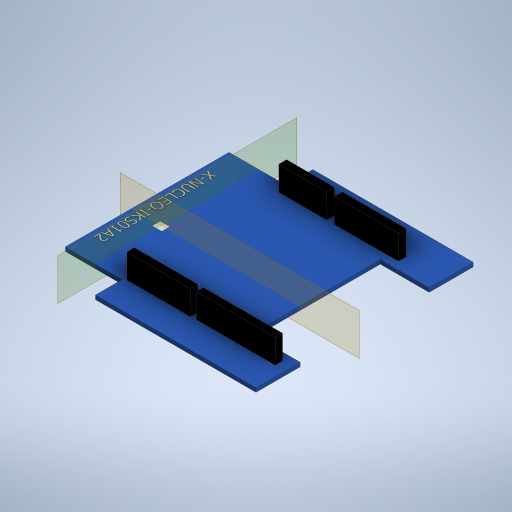
# Autodesk Inventor part: iks01A2base
Saved by Autodesk Inventor 2023 (Build 270158000, 158)
## iProperties
Created: 2023-11-05
Part Number: iks01A2base
Material: Générique
Document SubType Name: Modeling
Designer: eleves
Density: 1 g/cm^3
Appearance: Par défaut
Author: eleves
Autodesk Inventor part; units mm, degrees
ref_plane "YZ Plane" through (0, 0, 0) normal (1, 0, 0) x (0, 1, 0)
ref_plane "XZ Plane" through (0, 0, 0) normal (0, 1, 0) x (-1, 0, 0)
ref_plane "XY Plane" through (0, 0, 0) normal (0, 0, 1) x (1, 0, 0)
sketch "Esquisse1" plane through (0, 0, 0) normal (0, 1, 0) x (-1, 0, 0)
  line L0 (0, 0) -> (78.9893, 0) construction
  line L1 (78.9893, 0) -> (78.9893, -72.281) construction
  line L2 (78.9893, -72.281) -> (0, -72.281) construction
  line L3 (0, -72.281) -> (0, 0) construction
  line L4 (3.8993, -1.7198) -> (2.5066, -1.7198) construction
  line L5 (2.8077, -2.807) -> (2.8077, -1.7198) construction
  line L6 (53.7875, -2.8913) -> (53.7875, -1.7198) construction
  line L7 (53.7875, -1.7198) -> (2.8077, -1.7198) construction
  line L8 (70.571, -10.1894) -> (53.7875, -10.1894) construction
  line L9 (53.7875, -10.1894) -> (53.7875, -1.7198) construction
  line L10 (71.8197, -11.4429) -> (71.8197, -10.1894) construction
  line L11 (71.8197, -10.1894) -> (70.571, -10.1894) construction
  line L12 (71.8197, -10.1894) -> (71.8197, -40.9332) construction
  line L13 (4.0671, -15.7216) -> (2.8077, -15.7216) construction
  line L14 (2.8077, -15.7216) -> (2.8077, -1.7198) construction
  line L15 (4.0671, -15.7216) -> (18.3716, -15.7216) construction
  line L16 (18.326, -19.1106) -> (18.326, -15.7216) construction
  line L17 (18.326, -19.1106) -> (18.326, -45.5089) construction
  line L18 (71.8197, -40.9332) -> (71.8197, -61.0049) construction
  line L19 (70.7314, -62.1766) -> (71.8197, -62.1766) construction
  line L20 (71.8197, -62.1766) -> (71.8197, -61.0049) construction
  line L21 (53.7875, -64.2718) -> (53.7875, -62.1766) construction
  line L22 (53.7875, -62.1766) -> (70.7314, -62.1766) construction
  line L23 (52.6166, -70.7298) -> (53.7875, -70.7298) construction
  line L24 (53.7875, -70.7298) -> (53.7875, -64.2718) construction
  line L25 (16.1382, -56.7226) -> (18.326, -56.7226) construction
  line L26 (18.326, -56.7226) -> (18.326, -45.5089) construction
  line L27 (16.1382, -56.7226) -> (2.8077, -56.7226) construction
  line L28 (52.6166, -70.7298) -> (2.8077, -70.7298) construction
  line L29 (2.8077, -70.7298) -> (2.8077, -56.7226) construction
  line L30 (53.7875, -1.7198) -> (53.7875, -10.1894)
  line L31 (53.7875, -10.1894) -> (71.8197, -10.1894)
  line L32 (71.8197, -10.1894) -> (71.8197, -62.1766)
  line L33 (71.8197, -62.1766) -> (53.7875, -62.1766)
  line L34 (53.7875, -62.1766) -> (53.7875, -70.7298)
  line L35 (53.7875, -70.7298) -> (2.8077, -70.7298)
  line L36 (2.8077, -70.7298) -> (2.8077, -56.7226)
  line L37 (2.8077, -56.7226) -> (18.326, -56.7226)
  line L38 (18.326, -56.7226) -> (18.326, -15.7216)
  line L39 (18.326, -15.7216) -> (2.8077, -15.7216)
  line L40 (2.8077, -15.7216) -> (2.8077, -1.7198)
  line L41 (2.8077, -1.7198) -> (53.7875, -1.7198)
  line L42 (63.8524, -29.7258) -> (60.7561, -29.7258)
  line L43 (60.7561, -29.7258) -> (60.7561, -32.3255)
  line L44 (60.7561, -32.3255) -> (63.8524, -32.3255)
  line L45 (63.8524, -32.3255) -> (63.8524, -29.7258)
  line L46 (5.9145, -13.2045) -> (30.9784, -13.2045)
  line L47 (30.9784, -13.2045) -> (30.9784, -10.944)
  line L48 (30.9784, -10.944) -> (5.9145, -10.944)
  line L49 (5.9145, -10.944) -> (5.9145, -13.2045)
  line L50 (32.8087, -13.2045) -> (52.9636, -13.2045)
  line L51 (52.9636, -13.2045) -> (52.9636, -10.8161)
  line L52 (52.9636, -10.8161) -> (32.8087, -10.8161)
  line L53 (32.8087, -10.8161) -> (32.8087, -13.2045)
  line L54 (37.7726, -59.0838) -> (52.9535, -59.0838)
  line L55 (52.9535, -59.0838) -> (52.9535, -61.5907)
  line L56 (52.9535, -61.5907) -> (37.7726, -61.5907)
  line L57 (37.7726, -61.5907) -> (37.7726, -59.0838)
  line L58 (35.2014, -59.0838) -> (14.9598, -59.0838)
  line L59 (14.9598, -59.0838) -> (14.9598, -61.5907)
  line L60 (14.9598, -61.5907) -> (35.2014, -61.5907)
  line L61 (35.2014, -61.5907) -> (35.2014, -59.0838)
  constraints: 118 end point, 19 perpendicular, 13 parallel, 11 horizontal, 11 point on line, 8 collinear, 3 vertical, 2 other
extrude "Extrusion2" add sketch "Esquisse1" along normal blind 1.3 contours L30 L31 L32 L33 L34 L35 L36 L37 L38 L39 L40 L41 | L45 L44 L43 L42 | L49 L48 L47 L46 | L53 L52 L51 L50 | L54 L55 L56 L57 | L61 L60 L59 L58
extrude "Extrusion3" add sketch "Esquisse1" along normal blind 9 contours L49 L48 L47 L46 | L53 L52 L51 L50 | L54 L55 L56 L57 | L61 L60 L59 L58
extrude "Extrusion4" add sketch "Esquisse1" along normal blind 1.3001 contours L45 L44 L43 L42
sketch "Esquisse2" plane through (0, 0, 0) normal (0, -1, 0) x (1, 0, 0)
  line L0 (-52.9636, -13.2045) -> (-52.9636, -10.8161) projected
  line L1 (-52.9636, -10.8161) -> (-32.8087, -10.8161) projected
  line L2 (-32.8087, -10.8161) -> (-32.8087, -13.2045) projected
  line L3 (-32.8087, -13.2045) -> (-52.9636, -13.2045) projected
  line L4 (-30.9784, -13.2045) -> (-30.9784, -10.944) projected
  line L5 (-30.9784, -10.944) -> (-5.9145, -10.944) projected
  line L6 (-5.9145, -10.944) -> (-5.9145, -13.2045) projected
  line L7 (-5.9145, -13.2045) -> (-30.9784, -13.2045) projected
  line L8 (-37.7726, -61.5907) -> (-52.9535, -61.5907) projected
  line L9 (-52.9535, -61.5907) -> (-52.9535, -59.0838) projected
  line L10 (-52.9535, -59.0838) -> (-37.7726, -59.0838) projected
  line L11 (-37.7726, -59.0838) -> (-37.7726, -61.5907) projected
  line L12 (-14.9598, -59.0838) -> (-14.9598, -61.5907) projected
  line L13 (-14.9598, -61.5907) -> (-35.2014, -61.5907) projected
  line L14 (-35.2014, -61.5907) -> (-35.2014, -59.0838) projected
  line L15 (-35.2014, -59.0838) -> (-14.9598, -59.0838) projected
  line L16 (-5.9145, -12.0742) -> (-52.9636, -12.0103) construction
  circle A0 centre (-7.2085, -12.0725) radius 0.5
  line L17 (-8.4118, -12.0708) -> (-55.4609, -12.0069) construction
  circle A1 centre (-9.7058, -12.0691) radius 0.5
  line L18 (-10.9091, -12.0674) -> (-57.9582, -12.0035) construction
  circle A2 centre (-12.2031, -12.0657) radius 0.5
  line L19 (-13.4064, -12.0641) -> (-60.4555, -12.0001) construction
  circle A3 centre (-14.7004, -12.0623) radius 0.5
  line L20 (-15.9037, -12.0607) -> (-62.9528, -11.9968) construction
  circle A4 centre (-17.1977, -12.0589) radius 0.5
  line L21 (-18.401, -12.0573) -> (-65.4501, -11.9934) construction
  circle A5 centre (-19.695, -12.0555) radius 0.5
  line L22 (-20.8983, -12.0539) -> (-67.9474, -11.99) construction
  circle A6 centre (-22.1923, -12.0521) radius 0.5
  line L23 (-23.3956, -12.0505) -> (-70.4447, -11.9866) construction
  circle A7 centre (-24.6896, -12.0487) radius 0.5
  line L24 (-25.8929, -12.0471) -> (-72.942, -11.9832) construction
  circle A8 centre (-27.1869, -12.0453) radius 0.5
  line L25 (-28.3902, -12.0437) -> (-75.4393, -11.9798) construction
  circle A9 centre (-29.6842, -12.0419) radius 0.5
  circle A10 centre (-34.1027, -12.0359) radius 0.5
  circle A11 centre (-36.5997, -12.0326) radius 0.5
  line L26 (-8.4115, -12.0708) -> (-55.4606, -12.0069) construction
  circle A12 centre (-39.0967, -12.0292) radius 0.5
  line L27 (-10.9085, -12.0674) -> (-57.9576, -12.0035) construction
  circle A13 centre (-41.5937, -12.0258) radius 0.5
  line L28 (-13.4055, -12.0641) -> (-60.4546, -12.0001) construction
  circle A14 centre (-44.0907, -12.0224) radius 0.5
  line L29 (-15.9025, -12.0607) -> (-62.9516, -11.9968) construction
  circle A15 centre (-46.5877, -12.019) radius 0.5
  line L30 (-18.3995, -12.0573) -> (-65.4486, -11.9934) construction
  circle A16 centre (-49.0847, -12.0156) radius 0.5
  line L31 (-20.8965, -12.0539) -> (-67.9456, -11.99) construction
  circle A17 centre (-51.5817, -12.0122) radius 0.5
  line L32 (-23.3935, -12.0505) -> (-70.4426, -11.9866) construction
  line L33 (-14.9598, -60.3373) -> (-52.9535, -60.3373) construction
  circle A18 centre (-16.2538, -60.3373) radius 0.5
  circle A19 centre (-18.7508, -60.3373) radius 0.5
  circle A20 centre (-21.2478, -60.3373) radius 0.5
  circle A21 centre (-23.7448, -60.3373) radius 0.5
  circle A22 centre (-26.2418, -60.3373) radius 0.5
  circle A23 centre (-28.7388, -60.3373) radius 0.5
  circle A24 centre (-31.2358, -60.3373) radius 0.5
  circle A25 centre (-33.7328, -60.3373) radius 0.5
  circle A26 centre (-39.0666, -60.3373) radius 0.5
  circle A27 centre (-41.5636, -60.3373) radius 0.5
  circle A28 centre (-44.0606, -60.3373) radius 0.5
  circle A29 centre (-46.5576, -60.3373) radius 0.5
  circle A30 centre (-49.0546, -60.3373) radius 0.5
  circle A31 centre (-51.5516, -60.3373) radius 0.5
  point P0 (0, 0)
  point P1 (-9.7055, -12.0691)
  point P2 (-12.2025, -12.0657)
  point P3 (-14.6995, -12.0623)
  point P4 (-17.1965, -12.0589)
  point P5 (-19.6935, -12.0555)
  point P6 (-22.1905, -12.0521)
  point P7 (-24.6875, -12.0487)
  dimension "d16" = 1
  dimension "d17" = 1.294
  dimension "d20" = 2.4973
  dimension "d25" = 1
  dimension "d26" = 1.294
  dimension "d29" = 2.497
  dimension "d34" = 1.294
  dimension "d37" = 2.497
  dimension "d42" = 1
  dimension "d43" = 1
  dimension "d44" = 1.294
  dimension "d47" = 2.497
  constraints: 36 end point, 32 centre point, 20 point on line, 4 midpoint, 2 collinear, 2 horizontal, 111 other
  measures "d16" diameter of A0
  measures "d17" distance from line of L6 A0.centre
  measures "d20" distance of L16.start L17.start
  measures "d25" diameter of A10
  measures "d26" distance from line of L2 A10.centre
  measures "d29" distance of A10.centre A11.centre
  measures "d34" distance from line of L12 A18.centre
  measures "d37" distance of A18.centre A19.centre
  measures "d42" diameter of A18
  measures "d43" diameter of A26
  measures "d44" distance from line of L11 A26.centre
  measures "d47" distance of A26.centre A27.centre
extrude "Extrusion5" add sketch "Esquisse2" along normal blind 3 contours A0 | A1 | A2 | A3 | A4 | A5 | A6 | A7 | A8 | A9 | A10 | A11 | A12 | A13 | A14 | A15 | A16 | A17 | A18 | A19 | A20 | A21 | A22 | A23 | A24 | A25 | A26 | A27 | A28 | A29 | A30 | A31
sketch "Esquisse3" plane through (0, 1.3, 0) normal (0, 1, 0) x (1, 0, 0)
  line L0 (-66.9636, 53.8646) -> (-66.9636, 47.4032) construction
  line L1 (-66.9636, 47.4032) -> (-103.03, 47.4032) construction
  line L2 (-103.03, 47.4032) -> (-103.03, 53.8646) construction
  line L3 (-103.03, 53.8646) -> (-66.9636, 53.8646) construction
  line L4 (-70.0758, 51.4489) -> (-70.0758, 51.9133)
  line L5 (-70.0758, 51.9133) -> (-68.8606, 52.6543)
  line L6 (-68.8606, 52.6543) -> (-70.0758, 53.4101)
  line L7 (-70.0758, 53.4101) -> (-70.0758, 53.8473)
  line L8 (-70.0758, 53.8473) -> (-68.5494, 52.8766)
  line L9 (-68.5494, 52.8766) -> (-67.0278, 53.8177)
  line L10 (-67.0278, 53.8177) -> (-67.0278, 53.3533)
  line L11 (-67.0278, 53.3533) -> (-68.2209, 52.6271)
  line L12 (-68.2209, 52.6271) -> (-67.0278, 51.8861)
  line L13 (-67.0278, 51.8861) -> (-67.0278, 51.4489)
  line L14 (-67.0278, 51.4489) -> (-68.5296, 52.4024)
  line L15 (-68.5296, 52.4024) -> (-70.0758, 51.4489)
  line L16 (-68.9273, 50.0929) -> (-68.9273, 51.2464)
  line L17 (-68.9273, 51.2464) -> (-68.5568, 51.2464)
  line L18 (-68.5568, 51.2464) -> (-68.5568, 50.0929)
  line L19 (-68.5568, 50.0929) -> (-68.9273, 50.0929)
  line L20 (-70.0758, 47.4203) -> (-70.0758, 47.8748)
  line L21 (-70.0758, 47.8748) -> (-67.4478, 49.2234)
  line L22 (-67.4478, 49.2234) -> (-70.0758, 49.2234)
  line L23 (-70.0758, 49.2234) -> (-70.0758, 49.6014)
  line L24 (-70.0758, 49.6014) -> (-67.0278, 49.6014)
  line L25 (-67.0278, 49.6014) -> (-67.0278, 49.0258)
  line L26 (-67.0278, 49.0258) -> (-69.4411, 47.7982)
  line L27 (-69.4411, 47.7982) -> (-67.0278, 47.7982)
  line L28 (-67.0278, 47.7982) -> (-67.0278, 47.4203)
  line L29 (-67.0278, 47.4203) -> (-70.0758, 47.4203)
  spline S0 degree 2 poles (-70.1401, 45.7382) (-70.1401, 46.0075) (-69.9993, 46.4076) (-69.8585, 46.5484) knots 0 0 0 1 2 2 2
  spline S1 degree 2 poles (-69.8585, 46.5484) (-69.7004, 46.709) (-69.2558, 46.8399) (-68.9298, 46.8399) knots 0 0 0 1 2 2 2
  line L30 (-68.9298, 46.8399) -> (-67.0278, 46.8399)
  line L31 (-67.0278, 46.8399) -> (-67.0278, 46.4348)
  line L32 (-67.0278, 46.4348) -> (-68.9298, 46.4348)
  spline S2 degree 2 poles (-68.9298, 46.4348) (-69.1422, 46.4348) (-69.4287, 46.3805) (-69.5448, 46.3039) knots 0 0 0 1 2 2 2
  spline S3 degree 2 poles (-69.5448, 46.3039) (-69.6683, 46.2224) (-69.7943, 45.9408) (-69.7943, 45.7382) knots 0 0 0 1 2 2 2
  spline S4 degree 2 poles (-69.7943, 45.7382) (-69.7943, 45.5481) (-69.6683, 45.2517) (-69.5448, 45.1701) knots 0 0 0 1 2 2 2
  spline S5 degree 2 poles (-69.5448, 45.1701) (-69.4287, 45.0936) (-69.1447, 45.0392) (-68.9396, 45.0392) knots 0 0 0 1 2 2 2
  line L33 (-68.9396, 45.0392) -> (-67.0278, 45.0392)
  line L34 (-67.0278, 45.0392) -> (-67.0278, 44.6342)
  line L35 (-67.0278, 44.6342) -> (-68.9298, 44.6342)
  spline S6 degree 2 poles (-68.9298, 44.6342) (-69.2484, 44.6342) (-69.7029, 44.7626) (-69.8585, 44.9256) knots 0 0 0 1 2 2 2
  spline S7 degree 2 poles (-69.8585, 44.9256) (-70.0017, 45.0713) (-70.1401, 45.4567) (-70.1401, 45.7382) knots 0 0 0 1 2 2 2
  spline S8 degree 2 poles (-70.1302, 42.8632) (-70.1302, 43.1596) (-69.9301, 43.661) (-69.73, 43.8437) knots 0 0 0 1 2 2 2
  spline S9 degree 2 poles (-69.73, 43.8437) (-69.5324, 44.0265) (-68.9396, 44.2266) (-68.5543, 44.2266) knots 0 0 0 1 2 2 2
  spline S10 degree 2 poles (-68.5543, 44.2266) (-68.1715, 44.2266) (-67.6034, 44.0315) (-67.3934, 43.8462) knots 0 0 0 1 2 2 2
  spline S11 degree 2 poles (-67.3934, 43.8462) (-67.1884, 43.6634) (-66.9735, 43.1645) (-66.9735, 42.8557) knots 0 0 0 1 2 2 2
  spline S12 degree 2 poles (-66.9735, 42.8557) (-66.9735, 42.7026) (-67.018, 42.4334) (-67.0525, 42.3197) knots 0 0 0 1 2 2 2
  spline S13 degree 2 poles (-67.0525, 42.3197) (-67.0847, 42.2209) (-67.176, 42.0159) (-67.2304, 41.9147) knots 0 0 0 1 2 2 2
  line L36 (-67.2304, 41.9147) -> (-67.7195, 41.9147)
  line L37 (-67.7195, 41.9147) -> (-67.7195, 41.9468)
  spline S14 degree 2 poles (-67.7195, 41.9468) (-67.6701, 42.0011) (-67.5317, 42.1691) (-67.465, 42.2901) knots 0 0 0 1 2 2 2
  spline S15 degree 2 poles (-67.465, 42.2901) (-67.4008, 42.4062) (-67.3193, 42.6804) (-67.3193, 42.8582) knots 0 0 0 1 2 2 2
  spline S16 degree 2 poles (-67.3193, 42.8582) (-67.3193, 43.0533) (-67.4799, 43.4016) (-67.633, 43.5325) knots 0 0 0 1 2 2 2
  spline S17 degree 2 poles (-67.633, 43.5325) (-67.7886, 43.661) (-68.2604, 43.8042) (-68.5543, 43.8042) knots 0 0 0 1 2 2 2
  spline S18 degree 2 poles (-68.5543, 43.8042) (-68.868, 43.8042) (-69.32, 43.6536) (-69.4756, 43.5226) knots 0 0 0 1 2 2 2
  spline S19 degree 2 poles (-69.4756, 43.5226) (-69.6263, 43.3942) (-69.7794, 43.0509) (-69.7794, 42.8582) knots 0 0 0 1 2 2 2
  spline S20 degree 2 poles (-69.7794, 42.8582) (-69.7794, 42.6828) (-69.693, 42.384) (-69.6288, 42.2679) knots 0 0 0 1 2 2 2
  spline S21 degree 2 poles (-69.6288, 42.2679) (-69.5646, 42.1567) (-69.4312, 41.9912) (-69.3842, 41.9443) knots 0 0 0 1 2 2 2
  line L38 (-69.3842, 41.9443) -> (-69.3842, 41.9147)
  line L39 (-69.3842, 41.9147) -> (-69.8684, 41.9147)
  spline S22 degree 2 poles (-69.8684, 41.9147) (-69.9153, 42.0159) (-70.0017, 42.1938) (-70.0413, 42.3197) knots 0 0 0 1 2 2 2
  spline S23 degree 2 poles (-70.0413, 42.3197) (-70.0857, 42.4531) (-70.1302, 42.6804) (-70.1302, 42.8632) knots 0 0 0 1 2 2 2
  line L40 (-70.0758, 39.7707) -> (-70.0758, 41.5368)
  line L41 (-70.0758, 41.5368) -> (-67.0278, 41.5368)
  line L42 (-67.0278, 41.5368) -> (-67.0278, 41.1317)
  line L43 (-67.0278, 41.1317) -> (-69.7152, 41.1317)
  line L44 (-69.7152, 41.1317) -> (-69.7152, 39.7707)
  line L45 (-69.7152, 39.7707) -> (-70.0758, 39.7707)
  line L46 (-70.0758, 39.4521) -> (-67.0278, 39.4521)
  line L47 (-67.0278, 39.4521) -> (-67.0278, 37.5452)
  line L48 (-67.0278, 37.5452) -> (-67.3885, 37.5452)
  line L49 (-67.3885, 37.5452) -> (-67.3885, 39.047)
  line L50 (-67.3885, 39.047) -> (-68.2233, 39.047)
  line L51 (-68.2233, 39.047) -> (-68.2233, 37.6465)
  line L52 (-68.2233, 37.6465) -> (-68.584, 37.6465)
  line L53 (-68.584, 37.6465) -> (-68.584, 39.047)
  line L54 (-68.584, 39.047) -> (-69.7152, 39.047)
  line L55 (-69.7152, 39.047) -> (-69.7152, 37.5452)
  line L56 (-69.7152, 37.5452) -> (-70.0758, 37.5452)
  line L57 (-70.0758, 37.5452) -> (-70.0758, 39.4521)
  spline S24 degree 2 poles (-67.3761, 34.9443) (-67.5787, 34.7714) (-68.1715, 34.5787) (-68.5518, 34.5787) knots 0 0 0 1 2 2 2
  spline S25 degree 2 poles (-68.5518, 34.5787) (-68.9224, 34.5787) (-69.5226, 34.7664) (-69.7251, 34.9443) knots 0 0 0 1 2 2 2
  spline S26 degree 2 poles (-69.7251, 34.9443) (-69.9375, 35.132) (-70.1401, 35.6285) (-70.1401, 35.9273) knots 0 0 0 1 2 2 2
  spline S27 degree 2 poles (-70.1401, 35.9273) (-70.1401, 36.2361) (-69.9301, 36.7301) (-69.7251, 36.9104) knots 0 0 0 1 2 2 2
  spline S28 degree 2 poles (-69.7251, 36.9104) (-69.5226, 37.0858) (-68.9273, 37.2735) (-68.5518, 37.2735) knots 0 0 0 1 2 2 2
  spline S29 degree 2 poles (-68.5518, 37.2735) (-68.169, 37.2735) (-67.5861, 37.0833) (-67.3761, 36.9079) knots 0 0 0 1 2 2 2
  spline S30 degree 2 poles (-67.3761, 36.9079) (-67.1736, 36.7301) (-66.9636, 36.2336) (-66.9636, 35.9273) knots 0 0 0 1 2 2 2
  spline S31 degree 2 poles (-66.9636, 35.9273) (-66.9636, 35.6161) (-67.181, 35.1172) (-67.3761, 34.9443) knots 0 0 0 1 2 2 2
  spline S32 degree 2 poles (-68.5518, 35.0011) (-68.2505, 35.0011) (-67.7837, 35.132) (-67.6305, 35.2506) knots 0 0 0 1 2 2 2
  spline S33 degree 2 poles (-67.6305, 35.2506) (-67.4725, 35.3716) (-67.3144, 35.7125) (-67.3144, 35.9249) knots 0 0 0 1 2 2 2
  spline S34 degree 2 poles (-67.3144, 35.9249) (-67.3144, 36.1447) (-67.4675, 36.4757) (-67.6305, 36.6017) knots 0 0 0 1 2 2 2
  spline S35 degree 2 poles (-67.6305, 36.6017) (-67.7861, 36.7227) (-68.2554, 36.8511) (-68.5518, 36.8511) knots 0 0 0 1 2 2 2
  spline S36 degree 2 poles (-68.5518, 36.8511) (-69.1521, 36.8511) (-69.7893, 36.3472) (-69.7893, 35.9249) knots 0 0 0 1 2 2 2
  spline S37 degree 2 poles (-69.7893, 35.9249) (-69.7893, 35.5025) (-69.1521, 35.0011) (-68.5518, 35.0011) knots 0 0 0 1 2 2 2
  line L58 (-68.9273, 33.1041) -> (-68.9273, 34.2576)
  line L59 (-68.9273, 34.2576) -> (-68.5568, 34.2576)
  line L60 (-68.5568, 34.2576) -> (-68.5568, 33.1041)
  line L61 (-68.5568, 33.1041) -> (-68.9273, 33.1041)
  line L62 (-70.0758, 31.5505) -> (-70.0758, 32.7311)
  line L63 (-70.0758, 32.7311) -> (-69.7646, 32.7311)
  line L64 (-69.7646, 32.7311) -> (-69.7646, 32.3434)
  line L65 (-69.7646, 32.3434) -> (-67.3391, 32.3434)
  line L66 (-67.3391, 32.3434) -> (-67.3391, 32.7311)
  line L67 (-67.3391, 32.7311) -> (-67.0278, 32.7311)
  line L68 (-67.0278, 32.7311) -> (-67.0278, 31.5505)
  line L69 (-67.0278, 31.5505) -> (-67.3391, 31.5505)
  line L70 (-67.3391, 31.5505) -> (-67.3391, 31.9383)
  line L71 (-67.3391, 31.9383) -> (-69.7646, 31.9383)
  line L72 (-69.7646, 31.9383) -> (-69.7646, 31.5505)
  line L73 (-69.7646, 31.5505) -> (-70.0758, 31.5505)
  line L74 (-70.0758, 28.826) -> (-70.0758, 29.3522)
  line L75 (-70.0758, 29.3522) -> (-68.6581, 30.4661)
  line L76 (-68.6581, 30.4661) -> (-68.8581, 30.644)
  line L77 (-68.8581, 30.644) -> (-70.0758, 30.644)
  line L78 (-70.0758, 30.644) -> (-70.0758, 31.0491)
  line L79 (-70.0758, 31.0491) -> (-67.0278, 31.0491)
  line L80 (-67.0278, 31.0491) -> (-67.0278, 30.644)
  line L81 (-67.0278, 30.644) -> (-68.4283, 30.644)
  line L82 (-68.4283, 30.644) -> (-67.0278, 29.3942)
  line L83 (-67.0278, 29.3942) -> (-67.0278, 28.9001)
  line L84 (-67.0278, 28.9001) -> (-68.3888, 30.1623)
  line L85 (-68.3888, 30.1623) -> (-70.0758, 28.826)
  spline S38 degree 2 poles (-70.1302, 27.7343) (-70.1302, 28.0653) (-69.9919, 28.5296) (-69.8931, 28.7347) knots 0 0 0 1 2 2 2
  line L86 (-69.8931, 28.7347) -> (-69.3842, 28.7347)
  line L87 (-69.3842, 28.7347) -> (-69.3842, 28.705)
  spline S39 degree 2 poles (-69.3842, 28.705) (-69.572, 28.5049) (-69.7794, 27.9986) (-69.7794, 27.7639) knots 0 0 0 1 2 2 2
  spline S40 degree 2 poles (-69.7794, 27.7639) (-69.7794, 27.428) (-69.5003, 27.0847) (-69.2706, 27.0847) knots 0 0 0 1 2 2 2
  spline S41 degree 2 poles (-69.2706, 27.0847) (-69.0878, 27.0847) (-68.8606, 27.265) (-68.8038, 27.4601) knots 0 0 0 1 2 2 2
  spline S42 degree 2 poles (-68.8038, 27.4601) (-68.7643, 27.6009) (-68.7099, 27.8356) (-68.6655, 28.0109) knots 0 0 0 1 2 2 2
  spline S43 degree 2 poles (-68.6655, 28.0109) (-68.6235, 28.169) (-68.4975, 28.4185) (-68.3962, 28.5148) knots 0 0 0 1 2 2 2
  spline S44 degree 2 poles (-68.3962, 28.5148) (-68.295, 28.6087) (-68.0233, 28.7124) (-67.8454, 28.7124) knots 0 0 0 1 2 2 2
  spline S45 degree 2 poles (-67.8454, 28.7124) (-67.4749, 28.7124) (-66.9735, 28.1344) (-66.9735, 27.6874) knots 0 0 0 1 2 2 2
  spline S46 degree 2 poles (-66.9735, 27.6874) (-66.9735, 27.4305) (-67.0748, 26.976) (-67.1711, 26.7809) knots 0 0 0 1 2 2 2
  line L88 (-67.1711, 26.7809) -> (-67.6552, 26.7809)
  line L89 (-67.6552, 26.7809) -> (-67.6552, 26.8105)
  spline S47 degree 2 poles (-67.6552, 26.8105) (-67.5219, 26.9562) (-67.3242, 27.4107) (-67.3242, 27.6602) knots 0 0 0 1 2 2 2
  spline S48 degree 2 poles (-67.3242, 27.6602) (-67.3242, 27.9418) (-67.5885, 28.2901) (-67.8034, 28.2901) knots 0 0 0 1 2 2 2
  spline S49 degree 2 poles (-67.8034, 28.2901) (-67.9961, 28.2901) (-68.2258, 28.085) (-68.2777, 27.8924) knots 0 0 0 1 2 2 2
  spline S50 degree 2 poles (-68.2777, 27.8924) (-68.3123, 27.7639) (-68.4012, 27.391) (-68.4382, 27.2675) knots 0 0 0 1 2 2 2
  spline S51 degree 2 poles (-68.4382, 27.2675) (-68.5346, 26.9538) (-68.9224, 26.6623) (-69.2064, 26.6623) knots 0 0 0 1 2 2 2
  spline S52 degree 2 poles (-69.2064, 26.6623) (-69.3867, 26.6623) (-69.7325, 26.808) (-69.8535, 26.939) knots 0 0 0 1 2 2 2
  spline S53 degree 2 poles (-69.8535, 26.939) (-69.9869, 27.0847) (-70.1302, 27.4552) (-70.1302, 27.7343) knots 0 0 0 1 2 2 2
  spline S54 degree 2 poles (-68.5518, 24.4393) (-69.3719, 24.4393) (-70.1401, 24.916) (-70.1401, 25.4125) knots 0 0 0 1 2 2 2
  spline S55 degree 2 poles (-70.1401, 25.4125) (-70.1401, 25.9164) (-69.3571, 26.3881) (-68.5543, 26.3881) knots 0 0 0 1 2 2 2
  spline S56 degree 2 poles (-68.5543, 26.3881) (-67.7293, 26.3881) (-66.9661, 25.9114) (-66.9661, 25.4125) knots 0 0 0 1 2 2 2
  spline S57 degree 2 poles (-66.9661, 25.4125) (-66.9661, 24.9111) (-67.7565, 24.4393) (-68.5518, 24.4393) knots 0 0 0 1 2 2 2
  spline S58 degree 2 poles (-69.4806, 24.9629) (-69.3299, 24.9037) (-68.8655, 24.8543) (-68.5518, 24.8543) knots 0 0 0 1 2 2 2
  spline S59 degree 2 poles (-68.5518, 24.8543) (-68.2382, 24.8543) (-67.7763, 24.9037) (-67.6207, 24.9654) knots 0 0 0 1 2 2 2
  spline S60 degree 2 poles (-67.6207, 24.9654) (-67.465, 25.0272) (-67.3045, 25.2421) (-67.3045, 25.4125) knots 0 0 0 1 2 2 2
  spline S61 degree 2 poles (-67.3045, 25.4125) (-67.3045, 25.5829) (-67.465, 25.8027) (-67.6256, 25.867) knots 0 0 0 1 2 2 2
  spline S62 degree 2 poles (-67.6256, 25.867) (-67.7812, 25.9287) (-68.2554, 25.9732) (-68.5543, 25.9732) knots 0 0 0 1 2 2 2
  spline S63 degree 2 poles (-68.5543, 25.9732) (-68.8754, 25.9732) (-69.3052, 25.9337) (-69.4732, 25.8694) knots 0 0 0 1 2 2 2
  spline S64 degree 2 poles (-69.4732, 25.8694) (-69.6312, 25.8102) (-69.8017, 25.5903) (-69.8017, 25.4125) knots 0 0 0 1 2 2 2
  spline S65 degree 2 poles (-69.8017, 25.4125) (-69.8017, 25.2445) (-69.6411, 25.0247) (-69.4806, 24.9629) knots 0 0 0 1 2 2 2
  line L90 (-70.0758, 22.3225) -> (-70.0758, 23.8094)
  line L91 (-70.0758, 23.8094) -> (-69.7646, 23.8094)
  line L92 (-69.7646, 23.8094) -> (-69.7646, 23.2562)
  line L93 (-69.7646, 23.2562) -> (-67.7219, 23.2562)
  line L94 (-67.7219, 23.2562) -> (-67.7219, 23.8094)
  line L95 (-67.7219, 23.8094) -> (-67.4428, 23.8094)
  spline S66 degree 2 poles (-67.4428, 23.8094) (-67.4428, 23.4958) (-67.265, 23.1994) (-67.018, 23.1796) knots 0 0 0 1 2 2 2
  line L96 (-67.018, 23.1796) -> (-67.018, 22.8634)
  line L97 (-67.018, 22.8634) -> (-69.7646, 22.8634)
  line L98 (-69.7646, 22.8634) -> (-69.7646, 22.3225)
  line L99 (-69.7646, 22.3225) -> (-70.0758, 22.3225)
  line L100 (-70.0758, 22.0039) -> (-67.0278, 20.9763)
  line L101 (-67.0278, 20.9763) -> (-67.0278, 20.4774)
  line L102 (-67.0278, 20.4774) -> (-70.0758, 19.4499)
  line L103 (-70.0758, 19.4499) -> (-70.0758, 19.8772)
  line L104 (-70.0758, 19.8772) -> (-69.2237, 20.1538)
  line L105 (-69.2237, 20.1538) -> (-69.2237, 21.3172)
  line L106 (-69.2237, 21.3172) -> (-70.0758, 21.5938)
  line L107 (-70.0758, 21.5938) -> (-70.0758, 22.0039)
  line L108 (-68.8779, 20.265) -> (-67.4428, 20.7367)
  line L109 (-67.4428, 20.7367) -> (-68.8779, 21.206)
  line L110 (-68.8779, 21.206) -> (-68.8779, 20.265)
  line L111 (-70.0758, 17.3676) -> (-70.0758, 19.2473)
  line L112 (-70.0758, 19.2473) -> (-69.6436, 19.2473)
  spline S67 degree 2 poles (-69.6436, 19.2473) (-69.4534, 19.0448) (-69.1002, 18.6842) (-68.91, 18.5113) knots 0 0 0 1 2 2 2
  spline S68 degree 2 poles (-68.91, 18.5113) (-68.5271, 18.163) (-68.0677, 17.9086) (-67.8232, 17.9086) knots 0 0 0 1 2 2 2
  spline S69 degree 2 poles (-67.8232, 17.9086) (-67.6948, 17.9086) (-67.5021, 17.9876) (-67.4403, 18.0592) knots 0 0 0 1 2 2 2
  spline S70 degree 2 poles (-67.4403, 18.0592) (-67.3786, 18.1309) (-67.3168, 18.3186) (-67.3168, 18.4322) knots 0 0 0 1 2 2 2
  spline S71 degree 2 poles (-67.3168, 18.4322) (-67.3168, 18.5409) (-67.3712, 18.7632) (-67.4132, 18.8645) knots 0 0 0 1 2 2 2
  spline S72 degree 2 poles (-67.4132, 18.8645) (-67.4478, 18.9509) (-67.5466, 19.1115) (-67.5811, 19.1609) knots 0 0 0 1 2 2 2
  line L113 (-67.5811, 19.1609) -> (-67.5811, 19.1831)
  line L114 (-67.5811, 19.1831) -> (-67.1464, 19.1831)
  spline S73 degree 2 poles (-67.1464, 19.1831) (-67.0847, 19.0571) (-66.9636, 18.6051) (-66.9636, 18.4026) knots 0 0 0 1 2 2 2
  spline S74 degree 2 poles (-66.9636, 18.4026) (-66.9636, 17.9753) (-67.4156, 17.4936) (-67.801, 17.4936) knots 0 0 0 1 2 2 2
  spline S75 degree 2 poles (-67.801, 17.4936) (-67.9813, 17.4936) (-68.2826, 17.5776) (-68.4111, 17.6517) knots 0 0 0 1 2 2 2
  spline S76 degree 2 poles (-68.4111, 17.6517) (-68.5444, 17.7258) (-68.8063, 17.9407) (-68.9322, 18.0592) knots 0 0 0 1 2 2 2
  spline S77 degree 2 poles (-68.9322, 18.0592) (-69.1422, 18.2519) (-69.5917, 18.7237) (-69.7226, 18.8645) knots 0 0 0 1 2 2 2
  line L115 (-69.7226, 18.8645) -> (-69.7226, 17.3676)
  line L116 (-69.7226, 17.3676) -> (-70.0758, 17.3676)
  point P0 (0, 0)
  constraints: 2 other
extrude "Extrusion6" add sketch "Esquisse3" along normal blind 0.1
ref_plane "Plan de construction1" through (-62.3042, 1.3, -32.3255) normal (-1, 0, 0) x (0, 0, 1)
ref_plane "Plan de construction2" through (-63.8524, 1.3, -31.0257) normal (0, 0, 1) x (1, 0, 0)
